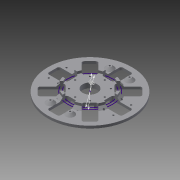
# Autodesk Inventor part: BaseArm
Saved by Autodesk Inventor 2015 (Build 190159000, 159)
## iProperties
Created: 2016-10-22
Part Number: BaseArm
Material: Generic
Document SubType Name: Modeling
Designer: Bardo91
Density: 1 g/cm^3
Appearance: Default
Author: Bardo91
Autodesk Inventor part; units mm, degrees
ref_plane "YZ Plane" through (0, 0, 0) normal (1, 0, 0) x (0, 1, 0)
ref_plane "XZ Plane" through (0, 0, 0) normal (0, 1, 0) x (-1, 0, 0)
ref_plane "XY Plane" through (0, 0, 0) normal (0, 0, 1) x (1, 0, 0)
sketch "Sketch1" plane through (0, 0, 0) normal (0, 0, 1) x (1, 0, 0)
  circle A0 centre (0, 0) radius 85
  dimension "d0" = 170
  constraints: 1 centre point, 1 coincident
  measures "d0" diameter of A0
extrude "Extrusion1" add sketch "Sketch1" along normal blind 5
sketch "Sketch2" plane through (0, 0, 5) normal (0, 0, 1) x (1, 0, 0)
  circle A0 centre (0, 0) radius 40
  circle A1 centre (0, 0) radius 45
  dimension "d3" = 80
  dimension "d4" = 90
  constraints: 2 centre point, 2 coincident
  measures "d3" diameter of A0
  measures "d4" diameter of A1
extrude "Extrusion2" add sketch "Sketch2" along normal blind 5 contours A0
extrude "Extrusion3" add sketch "Sketch2" along normal blind 10
sketch "Sketch4" plane through (0, 0, 10) normal (0, 0, 1) x (1, 0, 0)
  circle A0 centre (0, 0) radius 30
  circle A1 centre (0, 30) radius 1.75
  circle A2 centre (-21.2132, 21.2132) radius 1.75
  circle A3 centre (-30, 0) radius 1.75
  circle A4 centre (-21.2132, -21.2132) radius 1.75
  circle A5 centre (0, -30) radius 1.75
  circle A6 centre (21.2132, -21.2132) radius 1.75
  circle A7 centre (30, 0) radius 1.75
  circle A8 centre (21.2132, 21.2132) radius 1.75
  dimension "d12" = 60
  dimension "d13" = 3.5
  dimension "d16" = 360
  constraints: 8 centre point, 3 coincident, 1 vertical alignment, 25 other
  measures "d13" diameter of A1
extrude "Extrusion5" cut sketch "Sketch4" against normal through all contours A0 A7 | A0 A7 | A8 A0 | A0 A8 | A6 A0 | A0 A6 | A1 A0 | A0 A1 | A5 A0 | A0 A5 | A2 A0 | A0 A2 | A4 A0 | A0 A4 | A3 A0 | A0 A3
chamfer "Chamfer1" distance 5 angle 45 1 edges at (-45, 0, 5)
sketch "Sketch5" plane through (0, 0, 5) normal (0, 0, 1) x (1, 0, 0)
  line L0 (0, 0) -> (65.3, 0)
  line L1 (65.3, 0) -> (65.3, -18)
  line L2 (65.3, -18) -> (46.3, -18)
  line L3 (46.3, -18) -> (46.3, 18)
  line L4 (46.3, 18) -> (65.3, 18)
  line L5 (0, 0) -> (0, -32.4581)
  circle A0 centre (65.3, -18) radius 1.75
  circle A1 centre (46.3, -18) radius 1.75
  circle A2 centre (46.3, 18) radius 1.75
  circle A3 centre (65.3, 18) radius 1.75
  line L6 (0, 0) -> (-65.3, 0)
  line L7 (-65.3, 0) -> (-65.3, -18)
  line L8 (-65.3, -18) -> (-46.3, -18)
  line L9 (-46.3, -18) -> (-46.3, 18)
  line L10 (-46.3, 18) -> (-65.3, 18)
  circle A4 centre (-65.3, -18) radius 1.75
  circle A5 centre (-46.3, -18) radius 1.75
  circle A6 centre (-46.3, 18) radius 1.75
  circle A7 centre (-65.3, 18) radius 1.75
  dimension "d23" = 65.3
  dimension "d24" = 18
  dimension "d25" = 19
  dimension "d26" = 36
  dimension "d27" = 3.5
  dimension "d28" = 3.5
  dimension "d29" = 3.5
  dimension "d30" = 3.5
  constraints: 22 end point, 9 symmetric about line, 8 centre point, 8 coincident, 2 horizontal, 2 perpendicular, 2 vertical, 4 other
  measures "d23" distance of L0.start L0.end
  measures "d24" distance of L0.end L1.end
  measures "d25" distance of L1.end L2.end
  measures "d26" distance of L2.end L3.end
  measures "d27" diameter of A0
  measures "d28" diameter of A1
  measures "d29" diameter of A2
  measures "d30" diameter of A3
extrude "Extrusion6" cut sketch "Sketch5" along normal through all both and the other way through all contours A3 | A2 L4 L3 | L3 L4 A2 | A7 | A6 L10 L9 | L9 L10 A6 | A1 L2 L3 | L3 L2 A1 | A5 L8 L9 | L9 L8 A5 | A0 L2 L1 | L1 L2 A0 | A4 L8 L7 | L7 L8 A4
sketch "Sketch6" plane through (0, 0, 5) normal (0, 0, 1) x (1, 0, 0)
  point P0 (0, 0)
sketch "Sketch7" plane through (0, 0, 5) normal (0, 0, 1) x (1, 0, 0)
  line L0 (0, 0) -> (0, -40)
  line L1 (0, -40) -> (0, -60)
  line L2 (0, -60) -> (-20, -60)
  line L3 (-20, -60) -> (-20, -45)
  line L4 (-20, -45) -> (20, -45)
  line L5 (20, -45) -> (20, -60)
  circle A0 centre (20, -60) radius 1.75
  circle A1 centre (-20, -60) radius 1.75
  circle A2 centre (-20, -45) radius 1.75
  circle A3 centre (20, -45) radius 1.75
  circle A4 centre (20, -60) radius 3.5
  circle A5 centre (-20, -60) radius 3.5
  circle A6 centre (-20, -45) radius 3.5
  circle A7 centre (20, -45) radius 3.5
  line L6 (0, 0) -> (-50, 0)
  line L7 (0, 0) -> (0, 40)
  line L8 (0, 40) -> (0, 60)
  line L9 (0, 60) -> (-20, 60)
  line L10 (-20, 60) -> (-20, 45)
  line L11 (-20, 45) -> (20, 45)
  line L12 (20, 45) -> (20, 60)
  circle A8 centre (20, 60) radius 1.75
  circle A9 centre (-20, 60) radius 1.75
  circle A10 centre (-20, 45) radius 1.75
  circle A11 centre (20, 45) radius 1.75
  circle A12 centre (20, 60) radius 3.5
  circle A13 centre (-20, 60) radius 3.5
  circle A14 centre (-20, 45) radius 3.5
  circle A15 centre (20, 45) radius 3.5
  dimension "d33" = 40
  dimension "d34" = 20
  dimension "d35" = 20
  dimension "d36" = 15
  dimension "d37" = 40
  dimension "d38" = 3.5
  dimension "d39" = 3.5
  dimension "d40" = 3.5
  dimension "d41" = 3.5
  dimension "d42" = 7
  dimension "d43" = 7
  dimension "d44" = 7
  dimension "d45" = 7
  dimension "d46" = 50
  constraints: 26 end point, 16 centre point, 16 coincident, 14 symmetric about line, 3 perpendicular, 2 point on line, 2 vertical, 1 horizontal, 8 other
  measures "d33" distance of L0.start L0.end
  measures "d34" distance of L0.end L1.end
  measures "d35" distance of L1.end L2.end
  measures "d36" distance of L2.end L3.end
  measures "d37" distance of L3.end L4.end
  measures "d38" diameter of A0
  measures "d39" diameter of A1
  measures "d40" diameter of A2
  measures "d41" diameter of A3
  measures "d42" diameter of A4
  measures "d43" diameter of A5
  measures "d44" diameter of A6
  measures "d45" diameter of A7
  measures "d46" distance of L0.start L6.end
extrude "Extrusion7" add sketch "Sketch7" along normal blind 5 contours A4 | A12 | A5 L3 A1 L2 | L2 A1 L3 A5 | A13 L10 A9 L9 | L9 A9 L10 A13
extrude "Extrusion8" cut sketch "Sketch7" against normal through all contours A0 | A8 | A2 L3 L4 | L4 L3 A2 | A3 L5 L4 | L4 L5 A3 | A10 L10 L11 | L11 L10 A10 | A11 L12 L11 | L11 L12 A11 | A1 L3 L2 | L2 L3 A1 | A9 L10 L9 | L9 L10 A9
chamfer "Chamfer2" distance 5 angle 45 4 edges at (16.5, 60, 5) (-23.5, 60, 5) (-23.5, -60, 5) (16.5, -60, 5)
sketch "Sketch8" plane through (0, 0, 0) normal (0, 0, -1) x (-1, 0, 0)
  circle A0 centre (20, 60) radius 3.5 projected
  circle A1 centre (20, 60) radius 3.5
  circle A2 centre (20, 44.935) radius 3.5
  circle A3 centre (-19.9954, 45) radius 3.5
  circle A4 centre (-19.9954, 60) radius 3.5
  line L0 (0, 0) -> (32.9314, 0)
  circle A5 centre (20, -60) radius 3.5
  circle A6 centre (20, -60) radius 3.5
  circle A7 centre (20, -44.935) radius 3.5
  circle A8 centre (-19.9954, -45) radius 3.5
  circle A9 centre (-19.9954, -60) radius 3.5
  dimension "d54" = 7
  dimension "d55" = 7
  dimension "d56" = 7
  constraints: 9 centre point, 5 symmetric about line, 2 coincident, 2 end point, 1 horizontal, 5 other
  measures "d54" diameter of A2
  measures "d55" diameter of A3
  measures "d56" diameter of A4
extrude "Extrusion9" cut sketch "Sketch8" along normal mid plane 4
sketch "Sketch9" plane through (0, 0, 5) normal (0, 0, 1) x (1, 0, 0)
  line L0 (0, 0) -> (35, 0)
  line L1 (35, 0) -> (35, 8)
  line L2 (39, 12) -> (71, 12)
  line L3 (75, 8) -> (75, -8)
  line L4 (71, -12) -> (39, -12)
  line L5 (35, -8) -> (35, 0)
  arc A0 (71, -12) -> (75, -8) centre (71, -8) ccw
  arc A1 (75, 8) -> (71, 12) centre (71, 8) ccw
  arc A2 (39, 12) -> (35, 8) centre (39, 8) ccw
  arc A3 (35, -8) -> (39, -12) centre (39, -8) ccw
  line L6 (0, 0) -> (24.7487, 24.7487)
  line L7 (24.7487, 24.7487) -> (19.0919, 30.4056)
  line L8 (19.0919, 36.0624) -> (41.7193, 58.6899)
  line L9 (47.3762, 58.6899) -> (58.6899, 47.3762)
  line L10 (58.6899, 41.7193) -> (36.0624, 19.0919)
  line L11 (30.4056, 19.0919) -> (24.7487, 24.7487)
  arc A4 (58.6899, 41.7193) -> (58.6899, 47.3762) centre (55.8614, 44.5477) ccw
  arc A5 (47.3762, 58.6899) -> (41.7193, 58.6899) centre (44.5477, 55.8614) ccw
  arc A6 (19.0919, 36.0624) -> (19.0919, 30.4056) centre (21.9203, 33.234) ccw
  arc A7 (30.4056, 19.0919) -> (36.0624, 19.0919) centre (33.234, 21.9203) ccw
  line L12 (0, 0) -> (0, 35)
  line L13 (0, 35) -> (-8, 35)
  line L14 (-12, 39) -> (-12, 71)
  line L15 (-8, 75) -> (8, 75)
  line L16 (12, 71) -> (12, 39)
  line L17 (8, 35) -> (0, 35)
  arc A8 (12, 71) -> (8, 75) centre (8, 71) ccw
  arc A9 (-8, 75) -> (-12, 71) centre (-8, 71) ccw
  arc A10 (-12, 39) -> (-8, 35) centre (-8, 39) ccw
  arc A11 (8, 35) -> (12, 39) centre (8, 39) ccw
  line L18 (0, 0) -> (-24.7487, 24.7487)
  line L19 (-24.7487, 24.7487) -> (-30.4056, 19.0919)
  line L20 (-36.0624, 19.0919) -> (-58.6899, 41.7193)
  line L21 (-58.6899, 47.3762) -> (-47.3762, 58.6899)
  line L22 (-41.7193, 58.6899) -> (-19.0919, 36.0624)
  line L23 (-19.0919, 30.4056) -> (-24.7487, 24.7487)
  arc A12 (-41.7193, 58.6899) -> (-47.3762, 58.6899) centre (-44.5477, 55.8614) ccw
  arc A13 (-58.6899, 47.3762) -> (-58.6899, 41.7193) centre (-55.8614, 44.5477) ccw
  arc A14 (-36.0624, 19.0919) -> (-30.4056, 19.0919) centre (-33.234, 21.9203) ccw
  arc A15 (-19.0919, 30.4056) -> (-19.0919, 36.0624) centre (-21.9203, 33.234) ccw
  line L24 (0, 0) -> (-35, 0)
  line L25 (-35, 0) -> (-35, -8)
  line L26 (-39, -12) -> (-71, -12)
  line L27 (-75, -8) -> (-75, 8)
  line L28 (-71, 12) -> (-39, 12)
  line L29 (-35, 8) -> (-35, 0)
  arc A16 (-71, 12) -> (-75, 8) centre (-71, 8) ccw
  arc A17 (-75, -8) -> (-71, -12) centre (-71, -8) ccw
  arc A18 (-39, -12) -> (-35, -8) centre (-39, -8) ccw
  arc A19 (-35, 8) -> (-39, 12) centre (-39, 8) ccw
  line L30 (0, 0) -> (-24.7487, -24.7487)
  line L31 (-24.7487, -24.7487) -> (-19.0919, -30.4056)
  line L32 (-19.0919, -36.0624) -> (-41.7193, -58.6899)
  line L33 (-47.3762, -58.6899) -> (-58.6899, -47.3762)
  line L34 (-58.6899, -41.7193) -> (-36.0624, -19.0919)
  line L35 (-30.4056, -19.0919) -> (-24.7487, -24.7487)
  arc A20 (-58.6899, -41.7193) -> (-58.6899, -47.3762) centre (-55.8614, -44.5477) ccw
  arc A21 (-47.3762, -58.6899) -> (-41.7193, -58.6899) centre (-44.5477, -55.8614) ccw
  arc A22 (-19.0919, -36.0624) -> (-19.0919, -30.4056) centre (-21.9203, -33.234) ccw
  arc A23 (-30.4056, -19.0919) -> (-36.0624, -19.0919) centre (-33.234, -21.9203) ccw
  line L36 (0, 0) -> (0, -35)
  line L37 (0, -35) -> (8, -35)
  line L38 (12, -39) -> (12, -71)
  line L39 (8, -75) -> (-8, -75)
  line L40 (-12, -71) -> (-12, -39)
  line L41 (-8, -35) -> (0, -35)
  arc A24 (-12, -71) -> (-8, -75) centre (-8, -71) ccw
  arc A25 (8, -75) -> (12, -71) centre (8, -71) ccw
  arc A26 (12, -39) -> (8, -35) centre (8, -39) ccw
  arc A27 (-8, -35) -> (-12, -39) centre (-8, -39) ccw
  line L42 (0, 0) -> (24.7487, -24.7487)
  line L43 (24.7487, -24.7487) -> (30.4056, -19.0919)
  line L44 (36.0624, -19.0919) -> (58.6899, -41.7193)
  line L45 (58.6899, -47.3762) -> (47.3762, -58.6899)
  line L46 (41.7193, -58.6899) -> (19.0919, -36.0624)
  line L47 (19.0919, -30.4056) -> (24.7487, -24.7487)
  arc A28 (41.7193, -58.6899) -> (47.3762, -58.6899) centre (44.5477, -55.8614) ccw
  arc A29 (58.6899, -47.3762) -> (58.6899, -41.7193) centre (55.8614, -44.5477) ccw
  arc A30 (36.0624, -19.0919) -> (30.4056, -19.0919) centre (33.234, -21.9203) ccw
  arc A31 (19.0919, -30.4056) -> (19.0919, -36.0624) centre (21.9203, -33.234) ccw
  point P0 (35, 12)
  point P1 (75, 12)
  point P2 (75, -12)
  point P3 (35, -12)
  point P4 (16.2635, 33.234)
  point P5 (44.5477, 61.5183)
  point P6 (61.5183, 44.5477)
  point P7 (33.234, 16.2635)
  point P8 (-12, 35)
  point P9 (-12, 75)
  point P10 (12, 75)
  point P11 (12, 35)
  point P12 (-33.234, 16.2635)
  point P13 (-61.5183, 44.5477)
  point P14 (-44.5477, 61.5183)
  point P15 (-16.2635, 33.234)
  point P16 (-35, -12)
  point P17 (-75, -12)
  point P18 (-75, 12)
  point P19 (-35, 12)
  point P20 (-16.2635, -33.234)
  point P21 (-44.5477, -61.5183)
  point P22 (-61.5183, -44.5477)
  point P23 (-33.234, -16.2635)
  point P24 (12, -35)
  point P25 (12, -75)
  point P26 (-12, -75)
  point P27 (-12, -35)
  point P28 (33.234, -16.2635)
  point P29 (61.5183, -44.5477)
  point P30 (44.5477, -61.5183)
  point P31 (16.2635, -33.234)
  dimension "d59" = 35
  dimension "d60" = 12
  dimension "d61" = 40
  dimension "d62" = 24
  dimension "d63" = 4
  dimension "d66" = 360
  constraints: 96 end point, 72 point on line, 64 point on circle, 32 centre point, 8 tangent, 5 perpendicular, 3 equal radius, 2 coincident, 1 horizontal, 223 other
  measures "d59" distance of L0.start L0.end
  measures "d60" distance of L0.end point (35, 12)
  measures "d61" distance of point (35, 12) point (75, 12)
  measures "d62" distance of point (75, 12) point (75, -12)
  measures "d63" radius of A0
extrude "Extrusion10" cut sketch "Sketch9" along normal through all both and the other way through all
sketch "Sketch10" plane through (0, 0, 0) normal (0, 0, -1) x (-1, 0, 0)
  circle A0 centre (0, 0) radius 15
  dimension "d70" = 30
  constraints: 1 centre point, 1 coincident
  measures "d70" diameter of A0
extrude "Extrusion11" cut sketch "Sketch10" against normal through all
sketch "Sketch11" plane through (0, 0, 0) normal (0, 0, -1) x (-1, 0, 0)
  circle A0 centre (0, -30) radius 1.75 projected
  circle A1 centre (0, -30) radius 7.5
  circle A2 centre (21.2132, -21.2132) radius 7.5
  circle A3 centre (30, 0) radius 7.5
  circle A4 centre (21.2132, 21.2132) radius 7.5
  circle A5 centre (0, 30) radius 7.5
  circle A6 centre (-21.2132, 21.2132) radius 7.5
  circle A7 centre (-30, 0) radius 7.5
  circle A8 centre (-21.2132, -21.2132) radius 7.5
  point P0 (0, 0)
  dimension "d73" = 15
  dimension "d76" = 360
  constraints: 8 centre point, 1 coincident, 17 other
  measures "d73" diameter of A1
extrude "Extrusion12" cut sketch "Sketch11" against normal blind 5
body "Solid1"
